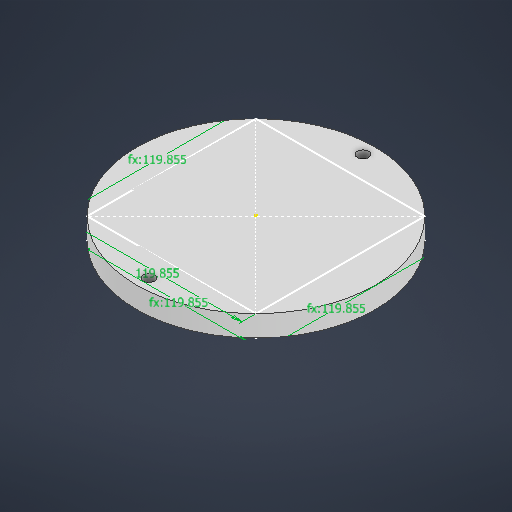
# Autodesk Inventor part: substrate plate
Saved by Autodesk Inventor 2026 (Build 300175050, 175E)
## iProperties
Created: 2024-06-21
Part Number: substrate plate
Material: Generic
Document SubType Name: Modeling
Designer: mayhe
Density: 1 g/cm^3
Appearance: Default
Author: mayhe
Autodesk Inventor part; units mm, degrees
ref_plane "YZ Plane" through (0, 0, 0) normal (1, 0, 0) x (0, 1, 0)
ref_plane "XZ Plane" through (0, 0, 0) normal (0, 1, 0) x (-1, 0, 0)
ref_plane "XY Plane" through (0, 0, 0) normal (0, 0, 1) x (1, 0, 0)
sketch "Sketch1" plane through (0, 0, 0) normal (0, 1, 0) x (-1, 0, 0)
  circle A0 centre (0, 0) radius 84.75
  dimension "d0" = 169.5
  constraints: 1 centre point, 1 coincident
  measures "d0" diameter of A0
extrude "Extrusion1" add sketch "Sketch1" along normal blind 15
sketch "Sketch2" plane through (0, 0, 0) normal (0, -1, 0) x (1, 0, 0)
  circle A0 centre (0, 0) radius 76
  circle A1 centre (0, 76) radius 4
  circle A2 centre (0, -76) radius 4
  circle A3 centre (0, 76) radius 2.25
  circle A4 centre (0, -76) radius 2.25
  dimension "d3" = 152
  dimension "d4" = 8
  dimension "d5" = 8
  dimension "d6" = 4.5
  dimension "d7" = 4.5
  constraints: 5 centre point, 3 point on circle, 2 coincident
  measures "d3" diameter of A0
  measures "d4" diameter of A1
  measures "d5" diameter of A2
  measures "d6" diameter of A3
  measures "d7" diameter of A4
extrude "Extrusion2" cut sketch "Sketch2" against normal through all contours A3 A0 | A0 A3 | A4 A0 | A0 A4
extrude "Extrusion3" cut sketch "Sketch2" against normal blind 12 contours A1 A0 A3 | A0 A3 A1 | A2 A0 A4 | A0 A4 A2 | A3 A0 | A0 A3 | A4 A0 | A0 A4
sketch "Sketch3" plane through (0, 0, 0) normal (0, -1, 0) x (1, 0, 0)
  line L0 (59.9273, 59.9273) -> (-59.9273, 59.9273)
  line L1 (-59.9273, 59.9273) -> (-59.9273, -59.9273)
  line L2 (-59.9273, -59.9273) -> (59.9273, -59.9273)
  line L3 (59.9273, -59.9273) -> (59.9273, 59.9273)
  line L4 (59.9273, 59.9273) -> (-59.9273, -59.9273) construction
  line L5 (-59.9273, 59.9273) -> (59.9273, -59.9273) construction
  point P0 (0, 0)
  dimension "d12" = 119.8546
  dimension "d13" = 119.8546
  constraints: 12 end point, 2 midpoint, 2 parallel, 1 horizontal, 1 perpendicular
  measures "d12" distance of L2.end L1.end
  measures "d13" distance of L1.end L0.end
sketch "Sketch4" plane through (0, 15, 0) normal (0, 1, 0) x (1, 0, 0)
  line L0 (-59.9273, -59.9273) -> (59.9273, -59.9273)
  line L1 (59.9273, -59.9273) -> (59.9273, 59.9273)
  line L2 (59.9273, 59.9273) -> (-59.9273, 59.9273)
  line L3 (-59.9273, 59.9273) -> (-59.9273, -59.9273)
  line L4 (-59.9273, -59.9273) -> (59.9273, 59.9273) construction
  line L5 (59.9273, -59.9273) -> (-59.9273, 59.9273) construction
  point P0 (0, 0)
  dimension "d14" = 119.8546
  dimension "d15" = 119.8546
  constraints: 12 end point, 2 midpoint, 2 parallel, 1 horizontal, 1 perpendicular
  measures "d14" distance of L1.end L2.end
  measures "d15" distance of L0.end L1.end
equation "\"d13\" = d12"
equation "\"d14\" = d12"
equation "\"d15\" = d12"
body "Solid1"
